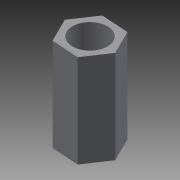
# Autodesk Inventor part: Arm Hex
Saved by Autodesk Inventor 2015 (Build 190159000, 159)
## iProperties
Created: 2015-02-17
Part Number: Arm Hex
Material: Generic
Document SubType Name: Modeling
Designer: chapale16
Density: 1 g/cm^3
Appearance: Default
Author: chapale16
Autodesk Inventor part; units mm, degrees
ref_plane "YZ Plane" through (0, 0, 0) normal (1, 0, 0) x (0, 1, 0)
ref_plane "XZ Plane" through (0, 0, 0) normal (0, 1, 0) x (-1, 0, 0)
ref_plane "XY Plane" through (0, 0, 0) normal (0, 0, 1) x (1, 0, 0)
sketch "Sketch1" plane through (0, 0, 0) normal (0, 1, 0) x (-1, 0, 0)
  line L0 (-4.0816, -6.1094) -> (-7.3317, 0.4801)
  line L1 (-7.3317, 0.4801) -> (-3.2501, 6.5895)
  line L2 (-3.2501, 6.5895) -> (4.0816, 6.1094)
  line L3 (4.0816, 6.1094) -> (7.3317, -0.4801)
  line L4 (7.3317, -0.4801) -> (3.2501, -6.5895)
  line L5 (3.2501, -6.5895) -> (-4.0816, -6.1094)
  circle A0 centre (0, 0) radius 4.7625
  dimension "d3" = 9.525
  constraints: 12 end point, 2 coincident, 1 centre point, 13 other
  measures "d3" diameter of A0
extrude "Extrusion2" add sketch "Sketch1" along normal blind 25.273
body "Solid2"
